Autodesk Inventor part; units mm, degrees
(part 2 of 3)
sketch "Эскиз4" plane through (0, 2, 0) normal (0, 1, 0) x (1, 0, 0)
  arc A0 (90.439454, -37.745267) -> (97.965347, -2.605931) centre (0, 0) ccw construction
  arc A1 (87.179537, -38.389169) -> (90.439454, -37.745267) centre (88.593751, -36.974956) ccw construction
  line L0 (87.179537, -38.389169) -> (83.085047, -34.294679) construction
  arc A2 (83.085047, -34.294679) -> (76.013979, -34.294679) centre (79.549513, -37.830213) ccw construction
  line L1 (76.013979, -34.294679) -> (67.882251, -42.426407) construction
  line L2 (67.882251, -42.426407) -> (47.125663, -21.669819) construction
  arc A3 (47.125663, -21.669819) -> (46.133514, -19.274559) centre (43.133514, -21.92031) ccw construction
  line L3 (46.133514, -19.274559) -> (46.133514, 19.274559) construction
  arc A4 (46.133514, 19.274559) -> (47.125663, 21.669819) centre (43.133514, 21.92031) ccw construction
  line L4 (47.125663, 21.669819) -> (67.882251, 42.426407) construction
  line L5 (67.882251, 42.426407) -> (76.013979, 34.294679) construction
  arc A5 (76.013979, 34.294679) -> (83.085047, 34.294679) centre (79.549513, 37.830213) ccw construction
  line L6 (83.085047, 34.294679) -> (87.179537, 38.389169) construction
  arc A6 (90.439454, 37.745267) -> (87.179537, 38.389169) centre (88.593751, 36.974956) ccw construction
  arc A7 (97.965347, 2.605931) -> (90.439454, 37.745267) centre (0, 0) ccw construction
  arc A8 (97.965347, 2.605931) -> (97.965347, -2.605931) centre (101, 0) ccw construction
  circle A9 centre (101, 0) radius 1.6 construction
  arc A10 (93.050296, -48.648149) -> (93.050296, 48.648149) centre (0, 0) ccw construction
  arc A11 (93.050296, 48.648149) -> (88.270396, 49.379523) centre (90.391716, 47.258202) ccw construction
  line L7 (88.270396, 49.379523) -> (85.206367, 46.315494) construction
  arc A12 (73.892659, 46.315494) -> (85.206367, 46.315494) centre (79.549513, 51.972348) ccw construction
  line L8 (73.892659, 46.315494) -> (46.315494, 73.892659) construction
  arc A13 (46.315494, 85.206367) -> (46.315494, 73.892659) centre (51.972348, 79.549513) ccw construction
  line L9 (46.315494, 85.206367) -> (49.379523, 88.270396) construction
  arc A14 (49.379523, 88.270396) -> (48.648149, 93.050296) centre (47.258202, 90.391716) ccw construction
  arc A15 (48.648149, 93.050296) -> (-48.648149, 93.050296) centre (0, 0) ccw construction
  arc A16 (-48.648149, 93.050296) -> (-49.379523, 88.270396) centre (-47.258202, 90.391716) ccw construction
  line L10 (-49.379523, 88.270396) -> (-46.315494, 85.206367) construction
  arc A17 (-46.315494, 73.892659) -> (-46.315494, 85.206367) centre (-51.972348, 79.549513) ccw construction
  line L11 (-46.315494, 73.892659) -> (-73.892659, 46.315494) construction
  arc A18 (-85.206367, 46.315494) -> (-73.892659, 46.315494) centre (-79.549513, 51.972348) ccw construction
  line L12 (-85.206367, 46.315494) -> (-88.270396, 49.379523) construction
  arc A19 (-88.270396, 49.379523) -> (-93.050296, 48.648149) centre (-90.391716, 47.258202) ccw construction
  arc A20 (-93.050296, 48.648149) -> (-93.050296, -48.648149) centre (0, 0) ccw construction
  arc A21 (-93.050296, -48.648149) -> (-88.270396, -49.379523) centre (-90.391716, -47.258202) ccw construction
  line L13 (-88.270396, -49.379523) -> (-85.206367, -46.315494) construction
  arc A22 (-73.892659, -46.315494) -> (-85.206367, -46.315494) centre (-79.549513, -51.972348) ccw construction
  line L14 (-73.892659, -46.315494) -> (-46.315494, -73.892659) construction
  arc A23 (-46.315494, -85.206367) -> (-46.315494, -73.892659) centre (-51.972348, -79.549513) ccw construction
  line L15 (-46.315494, -85.206367) -> (-49.379523, -88.270396) construction
  arc A24 (-49.379523, -88.270396) -> (-48.648149, -93.050296) centre (-47.258202, -90.391716) ccw construction
  arc A25 (-48.648149, -93.050296) -> (-45.41996, -94.667984) centre (0, 0) ccw construction
  arc A26 (-45.41996, -94.667984) -> (-43.035533, -94.165467) centre (-44.554817, -92.864785) ccw construction
  line L16 (-43.035533, -94.165467) -> (-18.380184, -65.366371) construction
  arc A27 (-17.477038, -64.764325) -> (-18.380184, -65.366371) centre (-16.8609, -66.667053) ccw construction
  line L17 (-17.477038, -64.764325) -> (-0.616138, -59.304458) construction
  arc A28 (0.616138, -59.304458) -> (-0.616138, -59.304458) centre (0, -61.207186) ccw construction
  line L18 (0.616138, -59.304458) -> (17.477038, -64.764325) construction
  arc A29 (18.380184, -65.366371) -> (17.477038, -64.764325) centre (16.8609, -66.667053) ccw construction
  line L19 (18.380184, -65.366371) -> (43.035533, -94.165467) construction
  arc A30 (43.035533, -94.165467) -> (45.41996, -94.667984) centre (44.554817, -92.864785) ccw construction
  arc A31 (45.41996, -94.667984) -> (48.648149, -93.050296) centre (0, 0) ccw construction
  arc A32 (48.648149, -93.050296) -> (49.379523, -88.270396) centre (47.258202, -90.391716) ccw construction
  line L20 (49.379523, -88.270396) -> (46.315494, -85.206367) construction
  arc A33 (46.315494, -73.892659) -> (46.315494, -85.206367) centre (51.972348, -79.549513) ccw construction
  line L21 (46.315494, -73.892659) -> (73.892659, -46.315494) construction
  arc A34 (85.206367, -46.315494) -> (73.892659, -46.315494) centre (79.549513, -51.972348) ccw construction
  line L22 (85.206367, -46.315494) -> (88.270396, -49.379523) construction
  arc A35 (88.270396, -49.379523) -> (93.050296, -48.648149) centre (90.391716, -47.258202) ccw construction
  circle A36 centre (-101, 0) radius 1.6 construction
  arc A37 (-90.439454, 37.745267) -> (-97.965347, 2.605931) centre (0, 0) ccw construction
  arc A38 (-87.179537, 38.389169) -> (-90.439454, 37.745267) centre (-88.593751, 36.974956) ccw construction
  line L23 (-87.179537, 38.389169) -> (-83.085047, 34.294679) construction
  arc A39 (-83.085047, 34.294679) -> (-76.013979, 34.294679) centre (-79.549513, 37.830213) ccw construction
  line L24 (-76.013979, 34.294679) -> (-67.882251, 42.426407) construction
  line L25 (-67.882251, 42.426407) -> (-47.125663, 21.669819) construction
  arc A40 (-47.125663, 21.669819) -> (-46.133514, 19.274559) centre (-43.133514, 21.92031) ccw construction
  line L26 (-46.133514, 19.274559) -> (-46.133514, -19.274559) construction
  arc A41 (-46.133514, -19.274559) -> (-47.125663, -21.669819) centre (-43.133514, -21.92031) ccw construction
  line L27 (-47.125663, -21.669819) -> (-67.882251, -42.426407) construction
  line L28 (-67.882251, -42.426407) -> (-76.013979, -34.294679) construction
  arc A42 (-76.013979, -34.294679) -> (-83.085047, -34.294679) centre (-79.549513, -37.830213) ccw construction
  line L29 (-83.085047, -34.294679) -> (-87.179537, -38.389169) construction
  arc A43 (-90.439454, -37.745267) -> (-87.179537, -38.389169) centre (-88.593751, -36.974956) ccw construction
  arc A44 (-97.965347, -2.605931) -> (-90.439454, -37.745267) centre (0, 0) ccw construction
  arc A45 (-97.965347, -2.605931) -> (-97.965347, 2.605931) centre (-101, 0) ccw construction
  circle A46 centre (45.111051, -90.365885) radius 1.6 construction
  circle A47 centre (45.111051, 90.365885) radius 1.6 construction
  circle A48 centre (90.365885, 45.111051) radius 1.6 construction
  circle A49 centre (-45.111051, -90.365885) radius 1.6 construction
  circle A50 centre (90.365885, -45.111051) radius 1.6 construction
  circle A51 centre (-45.111051, 90.365885) radius 1.6 construction
  circle A52 centre (-90.365885, 45.111051) radius 1.6 construction
  circle A53 centre (-90.365885, -45.111051) radius 1.6 construction
  line L30 (-63.63961, -46.669048) -> (-43.84062, -26.870058) construction
  arc A54 (-41.012193, -26.870058) -> (-43.84062, -26.870058) centre (-42.426407, -28.284271) ccw construction
  line L31 (-41.012193, -26.870058) -> (-26.870058, -41.012193) construction
  arc A55 (-26.870058, -43.84062) -> (-26.870058, -41.012193) centre (-28.284271, -42.426407) ccw construction
  line L32 (-26.870058, -43.84062) -> (-46.669048, -63.63961) construction
  line L33 (-46.669048, -63.63961) -> (-63.63961, -46.669048) construction
  line L34 (-42.426407, -67.882251) -> (-21.669819, -47.125663) construction
  arc A56 (-21.669819, -47.125663) -> (-19.274559, -46.133514) centre (-21.92031, -43.133514) ccw construction
  line L35 (-19.274559, -46.133514) -> (19.274559, -46.133514) construction
  arc A57 (19.274559, -46.133514) -> (21.669819, -47.125663) centre (21.92031, -43.133514) ccw construction
  line L36 (21.669819, -47.125663) -> (42.426407, -67.882251) construction
  line L37 (42.426407, -67.882251) -> (37.124381, -73.184277) construction
  arc A58 (34.190883, -73.070746) -> (37.124381, -73.184277) centre (35.710168, -71.770063) ccw construction
  line L38 (34.190883, -73.070746) -> (25.418693, -62.824241) construction
  arc A59 (24.841986, -61.889251) -> (25.418693, -62.824241) centre (28.115423, -60.51553) ccw construction
  line L39 (24.841986, -61.889251) -> (23.83128, -59.480842) construction
  arc A60 (23.83128, -59.480842) -> (21.004883, -57.332824) centre (20.557843, -60.854564) ccw construction
  line L40 (21.004883, -57.332824) -> (15.158499, -56.590699) construction
  arc A61 (14.511894, -56.446301) -> (15.158499, -56.590699) centre (15.605539, -53.068959) ccw construction
  line L41 (14.511894, -56.446301) -> (0.616138, -51.946601) construction
  arc A62 (0.616138, -51.946601) -> (-0.616138, -51.946601) centre (0, -53.849329) ccw construction
  line L42 (-0.616138, -51.946601) -> (-14.511894, -56.446301) construction
  arc A63 (-15.158499, -56.590699) -> (-14.511894, -56.446301) centre (-15.605539, -53.068959) ccw construction
  line L43 (-15.158499, -56.590699) -> (-21.004883, -57.332824) construction
  arc A64 (-21.004883, -57.332824) -> (-23.83128, -59.480842) centre (-20.557843, -60.854564) ccw construction
  line L44 (-23.83128, -59.480842) -> (-24.841986, -61.889251) construction
  arc A65 (-25.418693, -62.824241) -> (-24.841986, -61.889251) centre (-28.115423, -60.51553) ccw construction
  line L45 (-25.418693, -62.824241) -> (-34.190883, -73.070746) construction
  arc A66 (-37.124381, -73.184277) -> (-34.190883, -73.070746) centre (-35.710168, -71.770063) ccw construction
  line L46 (-37.124381, -73.184277) -> (-42.426407, -67.882251) construction
  line L47 (46.669048, -63.63961) -> (26.870058, -43.84062) construction
  arc A67 (26.870058, -41.012193) -> (26.870058, -43.84062) centre (28.284271, -42.426407) ccw construction
  line L48 (26.870058, -41.012193) -> (41.012193, -26.870058) construction
  arc A68 (43.84062, -26.870058) -> (41.012193, -26.870058) centre (42.426407, -28.284271) ccw construction
  line L49 (43.84062, -26.870058) -> (63.63961, -46.669048) construction
  line L50 (63.63961, -46.669048) -> (46.669048, -63.63961) construction
  line L51 (63.63961, 46.669048) -> (43.84062, 26.870058) construction
  arc A69 (41.012193, 26.870058) -> (43.84062, 26.870058) centre (42.426407, 28.284271) ccw construction
  line L52 (41.012193, 26.870058) -> (26.870058, 41.012193) construction
  arc A70 (26.870058, 43.84062) -> (26.870058, 41.012193) centre (28.284271, 42.426407) ccw construction
  line L53 (26.870058, 43.84062) -> (46.669048, 63.63961) construction
  line L54 (46.669048, 63.63961) -> (63.63961, 46.669048) construction
  line L55 (42.426407, 67.882251) -> (21.669819, 47.125663) construction
  arc A71 (21.669819, 47.125663) -> (19.274559, 46.133514) centre (21.92031, 43.133514) ccw construction
  line L56 (19.274559, 46.133514) -> (-19.274559, 46.133514) construction
  arc A72 (-19.274559, 46.133514) -> (-21.669819, 47.125663) centre (-21.92031, 43.133514) ccw construction
  line L57 (-21.669819, 47.125663) -> (-42.426407, 67.882251) construction
  line L58 (-42.426407, 67.882251) -> (-34.294679, 76.013979) construction
  arc A73 (-34.294679, 76.013979) -> (-34.294679, 83.085047) centre (-37.830213, 79.549513) ccw construction
  line L59 (-34.294679, 83.085047) -> (-38.389169, 87.179537) construction
  arc A74 (-37.745267, 90.439454) -> (-38.389169, 87.179537) centre (-36.974956, 88.593751) ccw construction
  arc A75 (37.745267, 90.439454) -> (-37.745267, 90.439454) centre (0, 0) ccw construction
  arc A76 (38.389169, 87.179537) -> (37.745267, 90.439454) centre (36.974956, 88.593751) ccw construction
  line L60 (38.389169, 87.179537) -> (34.294679, 83.085047) construction
  arc A77 (34.294679, 83.085047) -> (34.294679, 76.013979) centre (37.830213, 79.549513) ccw construction
  line L61 (34.294679, 76.013979) -> (42.426407, 67.882251) construction
  line L62 (-19.274559, 40.133514) -> (19.274559, 40.133514) construction
  arc A78 (19.274559, 40.133514) -> (21.669819, 39.141365) centre (21.92031, 43.133514) ccw construction
  line L63 (21.669819, 39.141365) -> (39.141365, 21.669819) construction
  arc A79 (39.141365, 21.669819) -> (40.133514, 19.274559) centre (43.133514, 21.92031) ccw construction
  line L64 (40.133514, 19.274559) -> (40.133514, -19.274559) construction
  arc A80 (40.133514, -19.274559) -> (39.141365, -21.669819) centre (43.133514, -21.92031) ccw construction
  line L65 (39.141365, -21.669819) -> (21.669819, -39.141365) construction
  arc A81 (21.669819, -39.141365) -> (19.274559, -40.133514) centre (21.92031, -43.133514) ccw construction
  line L66 (19.274559, -40.133514) -> (-19.274559, -40.133514) construction
  arc A82 (-19.274559, -40.133514) -> (-21.669819, -39.141365) centre (-21.92031, -43.133514) ccw construction
  line L67 (-21.669819, -39.141365) -> (-39.141365, -21.669819) construction
  arc A83 (-39.141365, -21.669819) -> (-40.133514, -19.274559) centre (-43.133514, -21.92031) ccw construction
  line L68 (-40.133514, -19.274559) -> (-40.133514, 19.274559) construction
  arc A84 (-40.133514, 19.274559) -> (-39.141365, 21.669819) centre (-43.133514, 21.92031) ccw construction
  line L69 (-39.141365, 21.669819) -> (-21.669819, 39.141365) construction
  arc A85 (-21.669819, 39.141365) -> (-19.274559, 40.133514) centre (-21.92031, 43.133514) ccw construction
  circle A86 centre (43.133514, 21.92031) radius 1.6 construction
  circle A87 centre (21.92031, -43.133514) radius 1.6 construction
  circle A88 centre (-21.92031, -43.133514) radius 1.6 construction
  circle A89 centre (-43.133514, -21.92031) radius 1.6 construction
  circle A90 centre (-43.133514, 21.92031) radius 1.6 construction
  circle A91 centre (-21.92031, 43.133514) radius 1.6 construction
  circle A92 centre (43.133514, -21.92031) radius 1.6 construction
  circle A93 centre (21.92031, 43.133514) radius 1.6 construction
  circle A94 centre (-37.830213, 79.549513) radius 1.6 construction
  circle A95 centre (-79.549513, 37.830213) radius 1.6 construction
  circle A96 centre (-79.549513, -37.830213) radius 1.6 construction
  circle A97 centre (79.549513, -37.830213) radius 1.6 construction
  circle A98 centre (37.830213, 79.549513) radius 1.6 construction
  circle A99 centre (79.549513, 37.830213) radius 1.6 construction
  circle A100 centre (-20.557843, -60.854564) radius 1.55 construction
  circle A101 centre (20.557843, -60.854564) radius 1.55 construction
  circle A102 centre (37.830213, -79.549513) radius 1.6 construction
  circle A103 centre (-37.830213, -79.549513) radius 1.6 construction
  line L70 (-46.669048, 63.63961) -> (-26.870058, 43.84062) construction
  arc A104 (-26.870058, 41.012193) -> (-26.870058, 43.84062) centre (-28.284271, 42.426407) ccw construction
  line L71 (-26.870058, 41.012193) -> (-41.012193, 26.870058) construction
  arc A105 (-43.84062, 26.870058) -> (-41.012193, 26.870058) centre (-42.426407, 28.284271) ccw construction
  line L72 (-43.84062, 26.870058) -> (-63.63961, 46.669048) construction
  line L73 (-63.63961, 46.669048) -> (-46.669048, 63.63961) construction
  circle A106 centre (0, 0) radius 101 construction
  circle A107 centre (-24, 98.107084) radius 1.6
  circle A108 centre (-24, 98.107084) radius 4
  line L74 (19.274559, 46.133514) -> (-19.274559, 46.133514) construction
  line L75 (0, 46.133514) -> (0, 40.133514) construction
  circle A109 centre (0, 46) radius 1.6
  arc A110 (-3.997771, 46.133514) -> (3.997771, 46.133514) centre (0, 46) ccw construction
  line L76 (-19.274559, 46.133514) -> (-6.25948, 46.133514) construction
  line L77 (6.25948, 46.133514) -> (19.274559, 46.133514) construction
  arc A111 (3.576846, 47.790579) -> (-3.576846, 47.790579) centre (0, 46) ccw
  arc A112 (-6.25948, 46.133514) -> (-3.576846, 47.790579) centre (-6.25948, 49.133514) ccw
  arc A113 (3.576846, 47.790579) -> (6.25948, 46.133514) centre (6.25948, 49.133514) ccw
  line L78 (6.25948, 46.133514) -> (6.25948, 42.111486)
  line L79 (6.25948, 42.111486) -> (-6.25948, 42.111486)
  line L80 (-6.25948, 42.111486) -> (-6.25948, 46.133514)
  line L81 (0, 0) -> (-30.405592, 30.405592) construction
  line L82 (-46.133514, -19.274559) -> (-46.133514, 19.274559) construction
  line L83 (-46.133514, -19.274559) -> (-46.133514, 19.274559) construction
  line L84 (-46.133514, 0) -> (-40.133514, 0) construction
  circle A114 centre (-46, 0) radius 1.6
  arc A115 (-46.133514, -3.997771) -> (-46.133514, 3.997771) centre (-46, 0) ccw construction
  line L85 (-46.133514, 19.274559) -> (-46.133514, 6.25948) construction
  line L86 (-46.133514, -6.25948) -> (-46.133514, -19.274559) construction
  arc A116 (-47.790579, 3.576846) -> (-47.790579, -3.576846) centre (-46, 0) ccw
  arc A117 (-47.790579, 3.576846) -> (-46.133514, 6.25948) centre (-49.133514, 6.25948) ccw
  arc A118 (-46.133514, -6.25948) -> (-47.790579, -3.576846) centre (-49.133514, -6.25948) ccw
  line L87 (-46.133514, -6.25948) -> (-42.111486, -6.25948)
  line L88 (-42.111486, -6.25948) -> (-42.111486, 6.25948)
  line L89 (-42.111486, 6.25948) -> (-46.133514, 6.25948)
  line L90 (0, 0) -> (0, -40.133514) construction
  line L91 (42.111486, 6.25948) -> (46.133514, 6.25948)
  line L92 (42.111486, -6.25948) -> (42.111486, 6.25948)
  arc A119 (46.133514, 6.25948) -> (47.790579, 3.576846) centre (49.133514, 6.25948) ccw
  arc A120 (47.790579, -3.576846) -> (47.790579, 3.576846) centre (46, 0) ccw
  arc A121 (47.790579, -3.576846) -> (46.133514, -6.25948) centre (49.133514, -6.25948) ccw
  line L93 (46.133514, -6.25948) -> (42.111486, -6.25948)
  circle A122 centre (46, 0) radius 1.6
  arc A123 (46.133514, 3.997771) -> (46.133514, -3.997771) centre (46, 0) ccw construction
  circle A124 centre (24, 98.107084) radius 1.6
  circle A125 centre (24, 98.107084) radius 4
  point P0 (46.133514, 0)
  point P1 (0, 101)
  dimension "d89" = 202
  dimension "d90" = 3.2
  dimension "d91" = 8
  dimension "d92" = 3.2
  dimension "d94" = 8
  dimension "d95" = 3
  dimension "d109" = 55
  dimension "d110" = 48
  constraints: 38 end point, 32 point on circle, 29 symmetric about line, 20 centre point, 11 point on line, 6 coincident, 4 midpoint, 4 tangent, 2 perpendicular, 1 collinear, 1 equal radius, 1 vertical, 12 other
  measures "d89" diameter of A106
  measures "d90" diameter of A107
  measures "d91" diameter of A108
  measures "d92" diameter of A109
  measures "d94" diameter of A110
  measures "d95" radius of A112
  measures "d109" distance of A106.end A109.centre
  measures "d110" distance of A124.centre A107.centre
extrude "Выдавливание5" cut sketch "Эскиз4" against normal blind 2 contours A107 | A109 | A114 | A122 | A124
extrude "Выдавливание6" add sketch "Эскиз4" against normal blind 2
sketch "Эскиз5" plane through (0, 2, 0) normal (0, 1, 0) x (1, 0, 0)
  circle A0 centre (-46, 0) radius 1.6 construction
  line L0 (-6.25948, 46.133514) -> (-19.274559, 46.133514) construction
  arc A1 (-19.274559, 46.133514) -> (-21.669819, 47.125663) centre (-21.92031, 43.133514) ccw construction
  line L1 (-21.669819, 47.125663) -> (-42.426407, 67.882251) construction
  line L2 (-42.426407, 67.882251) -> (-34.294679, 76.013979) construction
  arc A2 (-34.294679, 76.013979) -> (-34.294679, 83.085047) centre (-37.830213, 79.549513) ccw construction
  line L3 (-34.294679, 83.085047) -> (-38.389169, 87.179537) construction
  arc A3 (-37.745267, 90.439454) -> (-38.389169, 87.179537) centre (-36.974956, 88.593751) ccw construction
  arc A4 (-25.810185, 94.54012) -> (-37.745267, 90.439454) centre (0, 0) ccw construction
  arc A5 (-25.810185, 94.54012) -> (-20.747604, 95.778583) centre (-24, 98.107084) ccw construction
  arc A6 (20.747604, 95.778583) -> (-20.747604, 95.778583) centre (0, 0) ccw construction
  arc A7 (38.389169, 87.179537) -> (37.745267, 90.439454) centre (36.974956, 88.593751) ccw construction
  line L4 (38.389169, 87.179537) -> (34.294679, 83.085047) construction
  arc A8 (34.294679, 83.085047) -> (34.294679, 76.013979) centre (37.830213, 79.549513) ccw construction
  line L5 (34.294679, 76.013979) -> (42.426407, 67.882251) construction
  line L6 (42.426407, 67.882251) -> (21.669819, 47.125663) construction
  arc A9 (21.669819, 47.125663) -> (19.274559, 46.133514) centre (21.92031, 43.133514) ccw construction
  line L7 (19.274559, 46.133514) -> (6.25948, 46.133514) construction
  arc A10 (3.576846, 47.790579) -> (6.25948, 46.133514) centre (6.25948, 49.133514) ccw construction
  arc A11 (3.576846, 47.790579) -> (-3.576846, 47.790579) centre (0, 46) ccw construction
  arc A12 (-6.25948, 46.133514) -> (-3.576846, 47.790579) centre (-6.25948, 49.133514) ccw construction
  circle A13 centre (46, 0) radius 1.6 construction
  arc A14 (48.648149, 93.050296) -> (-48.648149, 93.050296) centre (0, 0) ccw construction
  arc A15 (-48.648149, 93.050296) -> (-49.379523, 88.270396) centre (-47.258202, 90.391716) ccw construction
  line L8 (-49.379523, 88.270396) -> (-46.315494, 85.206367) construction
  arc A16 (-46.315494, 73.892659) -> (-46.315494, 85.206367) centre (-51.972348, 79.549513) ccw construction
  line L9 (-46.315494, 73.892659) -> (-73.892659, 46.315494) construction
  arc A17 (-85.206367, 46.315494) -> (-73.892659, 46.315494) centre (-79.549513, 51.972348) ccw construction
  line L10 (-85.206367, 46.315494) -> (-88.270396, 49.379523) construction
  arc A18 (-88.270396, 49.379523) -> (-93.050296, 48.648149) centre (-90.391716, 47.258202) ccw construction
  arc A19 (-93.050296, 48.648149) -> (-93.050296, -48.648149) centre (0, 0) ccw construction
  arc A20 (-93.050296, -48.648149) -> (-88.270396, -49.379523) centre (-90.391716, -47.258202) ccw construction
  line L11 (-88.270396, -49.379523) -> (-85.206367, -46.315494) construction
  arc A21 (-73.892659, -46.315494) -> (-85.206367, -46.315494) centre (-79.549513, -51.972348) ccw construction
  line L12 (-73.892659, -46.315494) -> (-46.315494, -73.892659) construction
  arc A22 (-46.315494, -85.206367) -> (-46.315494, -73.892659) centre (-51.972348, -79.549513) ccw construction
  line L13 (-46.315494, -85.206367) -> (-49.379523, -88.270396) construction
  arc A23 (-49.379523, -88.270396) -> (-48.648149, -93.050296) centre (-47.258202, -90.391716) ccw construction
  arc A24 (-48.648149, -93.050296) -> (-45.41996, -94.667984) centre (0, 0) ccw construction
  arc A25 (-45.41996, -94.667984) -> (-43.035533, -94.165467) centre (-44.554817, -92.864785) ccw construction
  line L14 (-43.035533, -94.165467) -> (-18.380184, -65.366371) construction
  arc A26 (-17.477038, -64.764325) -> (-18.380184, -65.366371) centre (-16.8609, -66.667053) ccw construction
  line L15 (-17.477038, -64.764325) -> (-0.616138, -59.304458) construction
  arc A27 (0.616138, -59.304458) -> (-0.616138, -59.304458) centre (0, -61.207186) ccw construction
  line L16 (0.616138, -59.304458) -> (17.477038, -64.764325) construction
  arc A28 (18.380184, -65.366371) -> (17.477038, -64.764325) centre (16.8609, -66.667053) ccw construction
  line L17 (18.380184, -65.366371) -> (43.035533, -94.165467) construction
  arc A29 (43.035533, -94.165467) -> (45.41996, -94.667984) centre (44.554817, -92.864785) ccw construction
  arc A30 (45.41996, -94.667984) -> (48.648149, -93.050296) centre (0, 0) ccw construction
  arc A31 (48.648149, -93.050296) -> (49.379523, -88.270396) centre (47.258202, -90.391716) ccw construction
  line L18 (49.379523, -88.270396) -> (46.315494, -85.206367) construction
  arc A32 (46.315494, -73.892659) -> (46.315494, -85.206367) centre (51.972348, -79.549513) ccw construction
  line L19 (46.315494, -73.892659) -> (73.892659, -46.315494) construction
  arc A33 (85.206367, -46.315494) -> (73.892659, -46.315494) centre (79.549513, -51.972348) ccw construction
  line L20 (85.206367, -46.315494) -> (88.270396, -49.379523) construction
  arc A34 (88.270396, -49.379523) -> (93.050296, -48.648149) centre (90.391716, -47.258202) ccw construction
  arc A35 (93.050296, -48.648149) -> (93.050296, 48.648149) centre (0, 0) ccw construction
  arc A36 (93.050296, 48.648149) -> (88.270396, 49.379523) centre (90.391716, 47.258202) ccw construction
  line L21 (88.270396, 49.379523) -> (85.206367, 46.315494) construction
  arc A37 (73.892659, 46.315494) -> (85.206367, 46.315494) centre (79.549513, 51.972348) ccw construction
  line L22 (73.892659, 46.315494) -> (46.315494, 73.892659) construction
  arc A38 (46.315494, 85.206367) -> (46.315494, 73.892659) centre (51.972348, 79.549513) ccw construction
  line L23 (46.315494, 85.206367) -> (49.379523, 88.270396) construction
  arc A39 (49.379523, 88.270396) -> (48.648149, 93.050296) centre (47.258202, 90.391716) ccw construction
  circle A40 centre (-24, 98.107084) radius 1.6 construction
  circle A41 centre (0, 46) radius 1.6 construction
  arc A42 (47.790579, -3.576846) -> (46.133514, -6.25948) centre (49.133514, -6.25948) ccw construction
  arc A43 (47.790579, -3.576846) -> (47.790579, 3.576846) centre (46, 0) ccw construction
  arc A44 (46.133514, 6.25948) -> (47.790579, 3.576846) centre (49.133514, 6.25948) ccw construction
  line L24 (46.133514, 6.25948) -> (46.133514, 19.274559) construction
  arc A45 (46.133514, 19.274559) -> (47.125663, 21.669819) centre (43.133514, 21.92031) ccw construction
  line L25 (47.125663, 21.669819) -> (67.882251, 42.426407) construction
  line L26 (67.882251, 42.426407) -> (76.013979, 34.294679) construction
  arc A46 (76.013979, 34.294679) -> (83.085047, 34.294679) centre (79.549513, 37.830213) ccw construction
  line L27 (83.085047, 34.294679) -> (87.179537, 38.389169) construction
  arc A47 (90.439454, 37.745267) -> (87.179537, 38.389169) centre (88.593751, 36.974956) ccw construction
  arc A48 (97.965347, 2.605931) -> (90.439454, 37.745267) centre (0, 0) ccw construction
  arc A49 (97.965347, 2.605931) -> (97.965347, -2.605931) centre (101, 0) ccw construction
  arc A50 (90.439454, -37.745267) -> (97.965347, -2.605931) centre (0, 0) ccw construction
  arc A51 (87.179537, -38.389169) -> (90.439454, -37.745267) centre (88.593751, -36.974956) ccw construction
  line L28 (87.179537, -38.389169) -> (83.085047, -34.294679) construction
  arc A52 (83.085047, -34.294679) -> (76.013979, -34.294679) centre (79.549513, -37.830213) ccw construction
  line L29 (76.013979, -34.294679) -> (67.882251, -42.426407) construction
  line L30 (67.882251, -42.426407) -> (47.125663, -21.669819) construction
  arc A53 (47.125663, -21.669819) -> (46.133514, -19.274559) centre (43.133514, -21.92031) ccw construction
  line L31 (46.133514, -19.274559) -> (46.133514, -6.25948) construction
  circle A54 centre (101, 0) radius 1.6 construction
  circle A55 centre (-101, 0) radius 1.6 construction
  arc A56 (-47.790579, 3.576846) -> (-46.133514, 6.25948) centre (-49.133514, 6.25948) ccw construction
  arc A57 (-47.790579, 3.576846) -> (-47.790579, -3.576846) centre (-46, 0) ccw construction
  arc A58 (-46.133514, -6.25948) -> (-47.790579, -3.576846) centre (-49.133514, -6.25948) ccw construction
  line L32 (-46.133514, -6.25948) -> (-46.133514, -19.274559) construction
  arc A59 (-46.133514, -19.274559) -> (-47.125663, -21.669819) centre (-43.133514, -21.92031) ccw construction
  line L33 (-47.125663, -21.669819) -> (-67.882251, -42.426407) construction
  line L34 (-67.882251, -42.426407) -> (-76.013979, -34.294679) construction
  arc A60 (-76.013979, -34.294679) -> (-83.085047, -34.294679) centre (-79.549513, -37.830213) ccw construction
  line L35 (-83.085047, -34.294679) -> (-87.179537, -38.389169) construction
  arc A61 (-90.439454, -37.745267) -> (-87.179537, -38.389169) centre (-88.593751, -36.974956) ccw construction
  arc A62 (-97.965347, -2.605931) -> (-90.439454, -37.745267) centre (0, 0) ccw construction
  arc A63 (-97.965347, -2.605931) -> (-97.965347, 2.605931) centre (-101, 0) ccw construction
  arc A64 (-90.439454, 37.745267) -> (-97.965347, 2.605931) centre (0, 0) ccw construction
  arc A65 (-87.179537, 38.389169) -> (-90.439454, 37.745267) centre (-88.593751, 36.974956) ccw construction
  line L36 (-87.179537, 38.389169) -> (-83.085047, 34.294679) construction
  arc A66 (-83.085047, 34.294679) -> (-76.013979, 34.294679) centre (-79.549513, 37.830213) ccw construction
  line L37 (-76.013979, 34.294679) -> (-67.882251, 42.426407) construction
  line L38 (-67.882251, 42.426407) -> (-47.125663, 21.669819) construction
  arc A67 (-47.125663, 21.669819) -> (-46.133514, 19.274559) centre (-43.133514, 21.92031) ccw construction
  line L39 (-46.133514, 19.274559) -> (-46.133514, 6.25948) construction
  circle A68 centre (45.111051, -90.365885) radius 1.6 construction
  circle A69 centre (45.111051, 90.365885) radius 1.6 construction
  circle A70 centre (90.365885, 45.111051) radius 1.6 construction
  circle A71 centre (-45.111051, -90.365885) radius 1.6 construction
  circle A72 centre (90.365885, -45.111051) radius 1.6 construction
  circle A73 centre (-45.111051, 90.365885) radius 1.6 construction
  circle A74 centre (-90.365885, 45.111051) radius 1.6 construction
  circle A75 centre (-90.365885, -45.111051) radius 1.6 construction
  line L40 (-63.63961, -46.669048) -> (-43.84062, -26.870058) construction
  arc A76 (-41.012193, -26.870058) -> (-43.84062, -26.870058) centre (-42.426407, -28.284271) ccw construction
  line L41 (-41.012193, -26.870058) -> (-26.870058, -41.012193) construction
  arc A77 (-26.870058, -43.84062) -> (-26.870058, -41.012193) centre (-28.284271, -42.426407) ccw construction
  line L42 (-26.870058, -43.84062) -> (-46.669048, -63.63961) construction
  line L43 (-46.669048, -63.63961) -> (-63.63961, -46.669048) construction
  line L44 (-42.426407, -67.882251) -> (-21.669819, -47.125663) construction
  arc A78 (-21.669819, -47.125663) -> (-19.274559, -46.133514) centre (-21.92031, -43.133514) ccw construction
  line L45 (-19.274559, -46.133514) -> (19.274559, -46.133514) construction
  arc A79 (19.274559, -46.133514) -> (21.669819, -47.125663) centre (21.92031, -43.133514) ccw construction
  line L46 (21.669819, -47.125663) -> (42.426407, -67.882251) construction
  line L47 (42.426407, -67.882251) -> (37.124381, -73.184277) construction
  arc A80 (34.190883, -73.070746) -> (37.124381, -73.184277) centre (35.710168, -71.770063) ccw construction
  line L48 (34.190883, -73.070746) -> (25.418693, -62.824241) construction
  arc A81 (24.841986, -61.889251) -> (25.418693, -62.824241) centre (28.115423, -60.51553) ccw construction
  line L49 (24.841986, -61.889251) -> (23.83128, -59.480842) construction
  arc A82 (23.83128, -59.480842) -> (21.004883, -57.332824) centre (20.557843, -60.854564) ccw construction
  line L50 (21.004883, -57.332824) -> (15.158499, -56.590699) construction
  arc A83 (14.511894, -56.446301) -> (15.158499, -56.590699) centre (15.605539, -53.068959) ccw construction
  line L51 (14.511894, -56.446301) -> (0.616138, -51.946601) construction
  arc A84 (0.616138, -51.946601) -> (-0.616138, -51.946601) centre (0, -53.849329) ccw construction
  line L52 (-0.616138, -51.946601) -> (-14.511894, -56.446301) construction
  arc A85 (-15.158499, -56.590699) -> (-14.511894, -56.446301) centre (-15.605539, -53.068959) ccw construction
  line L53 (-15.158499, -56.590699) -> (-21.004883, -57.332824) construction
  arc A86 (-21.004883, -57.332824) -> (-23.83128, -59.480842) centre (-20.557843, -60.854564) ccw construction
  line L54 (-23.83128, -59.480842) -> (-24.841986, -61.889251) construction
  arc A87 (-25.418693, -62.824241) -> (-24.841986, -61.889251) centre (-28.115423, -60.51553) ccw construction
  line L55 (-25.418693, -62.824241) -> (-34.190883, -73.070746) construction
  arc A88 (-37.124381, -73.184277) -> (-34.190883, -73.070746) centre (-35.710168, -71.770063) ccw construction
  line L56 (-37.124381, -73.184277) -> (-42.426407, -67.882251) construction
  line L57 (46.669048, -63.63961) -> (26.870058, -43.84062) construction
  arc A89 (26.870058, -41.012193) -> (26.870058, -43.84062) centre (28.284271, -42.426407) ccw construction
  line L58 (26.870058, -41.012193) -> (41.012193, -26.870058) construction
  arc A90 (43.84062, -26.870058) -> (41.012193, -26.870058) centre (42.426407, -28.284271) ccw construction
  line L59 (43.84062, -26.870058) -> (63.63961, -46.669048) construction
  line L60 (63.63961, -46.669048) -> (46.669048, -63.63961) construction
  line L61 (63.63961, 46.669048) -> (43.84062, 26.870058) construction
  arc A91 (41.012193, 26.870058) -> (43.84062, 26.870058) centre (42.426407, 28.284271) ccw construction
  line L62 (41.012193, 26.870058) -> (26.870058, 41.012193) construction
  arc A92 (26.870058, 43.84062) -> (26.870058, 41.012193) centre (28.284271, 42.426407) ccw construction
  line L63 (26.870058, 43.84062) -> (46.669048, 63.63961) construction
  line L64 (46.669048, 63.63961) -> (63.63961, 46.669048) construction
  line L65 (-19.274559, 40.133514) -> (19.274559, 40.133514) construction
  arc A93 (19.274559, 40.133514) -> (21.669819, 39.141365) centre (21.92031, 43.133514) ccw construction
  line L66 (21.669819, 39.141365) -> (39.141365, 21.669819) construction
  arc A94 (39.141365, 21.669819) -> (40.133514, 19.274559) centre (43.133514, 21.92031) ccw construction
  line L67 (40.133514, 19.274559) -> (40.133514, -19.274559) construction
  arc A95 (40.133514, -19.274559) -> (39.141365, -21.669819) centre (43.133514, -21.92031) ccw construction
  line L68 (39.141365, -21.669819) -> (21.669819, -39.141365) construction
  arc A96 (21.669819, -39.141365) -> (19.274559, -40.133514) centre (21.92031, -43.133514) ccw construction
  line L69 (19.274559, -40.133514) -> (-19.274559, -40.133514) construction
  arc A97 (-19.274559, -40.133514) -> (-21.669819, -39.141365) centre (-21.92031, -43.133514) ccw construction
  line L70 (-21.669819, -39.141365) -> (-39.141365, -21.669819) construction
  arc A98 (-39.141365, -21.669819) -> (-40.133514, -19.274559) centre (-43.133514, -21.92031) ccw construction
  line L71 (-40.133514, -19.274559) -> (-40.133514, 19.274559) construction
  arc A99 (-40.133514, 19.274559) -> (-39.141365, 21.669819) centre (-43.133514, 21.92031) ccw construction
  line L72 (-39.141365, 21.669819) -> (-21.669819, 39.141365) construction
  arc A100 (-21.669819, 39.141365) -> (-19.274559, 40.133514) centre (-21.92031, 43.133514) ccw construction
  circle A101 centre (43.133514, 21.92031) radius 1.6 construction
  circle A102 centre (21.92031, -43.133514) radius 1.6 construction
  circle A103 centre (-21.92031, -43.133514) radius 1.6 construction
  circle A104 centre (-43.133514, -21.92031) radius 1.6 construction
  circle A105 centre (-43.133514, 21.92031) radius 1.6 construction
  circle A106 centre (-21.92031, 43.133514) radius 1.6 construction
  circle A107 centre (43.133514, -21.92031) radius 1.6 construction
  circle A108 centre (21.92031, 43.133514) radius 1.6 construction
  circle A109 centre (-37.830213, 79.549513) radius 1.6 construction
  circle A110 centre (-79.549513, 37.830213) radius 1.6 construction
  circle A111 centre (-79.549513, -37.830213) radius 1.6 construction
  circle A112 centre (79.549513, -37.830213) radius 1.6 construction
  circle A113 centre (37.830213, 79.549513) radius 1.6 construction
  circle A114 centre (79.549513, 37.830213) radius 1.6 construction
  circle A115 centre (-20.557843, -60.854564) radius 1.55 construction
  circle A116 centre (20.557843, -60.854564) radius 1.55 construction
  circle A117 centre (37.830213, -79.549513) radius 1.6 construction
  circle A118 centre (-37.830213, -79.549513) radius 1.6 construction
  line L73 (-46.669048, 63.63961) -> (-26.870058, 43.84062) construction
  arc A119 (-26.870058, 41.012193) -> (-26.870058, 43.84062) centre (-28.284271, 42.426407) ccw construction
  line L74 (-26.870058, 41.012193) -> (-41.012193, 26.870058) construction
  arc A120 (-43.84062, 26.870058) -> (-41.012193, 26.870058) centre (-42.426407, 28.284271) ccw construction
  line L75 (-43.84062, 26.870058) -> (-63.63961, 46.669048) construction
  line L76 (-63.63961, 46.669048) -> (-46.669048, 63.63961) construction
  circle A121 centre (0, -40) radius 1.6
  line L77 (0, -40.133514) -> (0, 0) construction
  arc A122 (0, -36) -> (-3.649244, -38.362008) centre (0, -40) ccw
  line L78 (19.274559, -40.133514) -> (6.386177, -40.133514) construction
  line L79 (19.274559, -40.133514) -> (-19.274559, -40.133514) construction
  line L80 (-6.386177, -40.133514) -> (-19.274559, -40.133514) construction
  arc A123 (3.649244, -38.362008) -> (0, -36) centre (0, -40) ccw
  arc A124 (-3.997771, -40.133514) -> (3.997771, -40.133514) centre (0, -40) ccw construction
  arc A125 (3.649244, -38.362008) -> (6.386177, -40.133514) centre (6.386177, -37.133514) ccw
  arc A126 (-6.386177, -40.133514) -> (-3.649244, -38.362008) centre (-6.386177, -37.133514) ccw
  line L81 (6.386177, -40.133514) -> (3.837324, -44.953044)
  line L82 (3.837324, -44.953044) -> (-3.266075, -45.278441)
  line L83 (-3.266075, -45.278441) -> (-6.386177, -40.133514)
  arc A127 (20.747604, 95.778583) -> (25.810185, 94.54012) centre (24, 98.107084) ccw
  arc A128 (37.745267, 90.439454) -> (25.810185, 94.54012) centre (0, 0) ccw
  dimension "d100" = 3.2
  dimension "d101" = 40
  dimension "d103" = 3
  dimension "d104" = 4
  constraints: 12 end point, 12 point on circle, 6 centre point, 6 point on line, 4 tangent, 1 coincident, 1 collinear, 1 equal radius, 1 midpoint, 1 vertical
  measures "d100" diameter of A121
  measures "d101" distance of point (0, 0) A121.centre
  measures "d103" radius of A125
  measures "d104" radius of A124
extrude "Выдавливание7" add sketch "Эскиз5" against normal blind 2
extrude "Выдавливание8" cut sketch "Эскиз5" against normal blind 2 contours A121